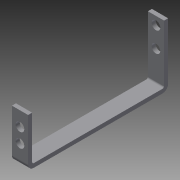
# Autodesk Inventor part: bottom pulley mount
Saved by Autodesk Inventor 2013 (Build 170138000, 138)
## iProperties
Created: 2013-02-07
Part Number: bottom pulley mount
Material: Generic
Document SubType Name: Sheet Metal
Designer: Arpan
Density: 1 g/cm^3
Sheet Metal Rule: Default
Mass: 7.12438 g
Surface Area: 60.3167 cm^2
Volume: 7.12438 cm^3
Author: Arpan
Autodesk Inventor part; units mm, degrees
ref_plane "YZ Plane" through (0, 0, 0) normal (1, 0, 0) x (0, 1, 0)
ref_plane "XZ Plane" through (0, 0, 0) normal (0, 1, 0) x (-1, 0, 0)
ref_plane "XY Plane" through (0, 0, 0) normal (0, 0, 1) x (1, 0, 0)
sketch "Sketch1" plane through (0, 0, 0) normal (0, 0, 1) x (1, 0, 0)
  line L0 (0, 0) -> (-12.7, 0)
  line L1 (-12.7, 0) -> (-12.7, 44.45)
  line L2 (-12.7, 44.45) -> (0, 44.45)
  line L3 (0, 44.45) -> (0, 0)
  dimension "d0" = 12.7
  dimension "d1" = 44.45
  measures "d0" distance of L0.start L0.end
  measures "d1" distance of L0.end L1.end
extrude "Plate1" add sketch "Sketch1" along normal blind 3.175
sketch "Sketch2" plane through (0, -1.27, 4.445) normal (0, -1, 0) x (1, 0, 0)
  line L0 (-12.7, 0) -> (0, 0)
  line L1 (0, 0) -> (0, 100.8952)
  line L2 (0, 100.8952) -> (-12.7, 100.8952)
  line L3 (-12.7, 100.8952) -> (-12.7, 0)
  constraints: 6 end point, 1 horizontal, 1 perpendicular, 1 vertical
edge flange "Flange1" height 105.3401 angle 90 thickness 3.175 bend radius 1.27 thickness toward (0, -1, 0) relief tear relief width 3.175 relief depth 1.5875 edges at (-6.35, 0, 3.175) wall of the first edge with corners at (-12.7, -1.27, 4.445) (0, -1.27, 4.445) (0, -1.27, 105.3401) (-12.7, -1.27, 105.3401)
bend "Bend1"
corner "Corner1"
sketch "Sketch3" plane through (0, 0, 0) normal (0, 0, -1) x (-1, 0, 0)
  circle A0 centre (6.3516, 38.1) radius 3.3782 projected
  circle A1 centre (6.3516, 22.225) radius 3.3782 projected
extrude "Cut1" cut sketch "Sketch3" against normal blind 3.175
sketch "Sketch5" plane through (0, 0, 106.6102) normal (0, 0, 1) x (1, 0, 0)
  line L0 (-12.7, 0) -> (0, 0)
  line L1 (0, 0) -> (0, 33.655)
  line L2 (0, 33.655) -> (-12.7, 33.655)
  line L3 (-12.7, 33.655) -> (-12.7, 0)
  constraints: 6 end point, 1 horizontal, 1 perpendicular, 1 vertical
edge flange "Flange2" height 38.1 angle 90 thickness 3.175 bend radius 1.27 thickness toward (0, 0, 1) relief tear relief width 3.175 relief depth 1.5875 edges at (-6.35, -1.27, 105.3401) wall of the first edge with corners at (-12.7, 0, 106.6102) (0, 0, 106.6102) (0, 33.655, 106.6102) (-12.7, 33.655, 106.6102)
bend "Bend2"
corner "Corner2"
sketch "Sketch6" plane through (-12.7, 33.655, 109.7851) normal (0, 0, 1) x (1, 0, 0)
  line L0 (0, 0) -> (12.7, 0) projected
  line L1 (0, -33.655) -> (0, 0) projected
  line L2 (6.35, 0) -> (6.35, -11.2183)
  line L3 (6.35, -11.2183) -> (6.35, -22.4451)
  circle A0 centre (6.35, -11.2183) radius 3.3782
  circle A1 centre (6.35, -22.4451) radius 3.3782
  dimension "d29" = 11.2183
  dimension "d31" = 11.2268
  dimension "d32" = 6.7564
  dimension "d33" = 6.7564
  constraints: 4 end point, 2 centre point, 2 coincident, 1 collinear, 1 midpoint, 1 parallel
  measures "d29" distance of L2.start L2.end
  measures "d31" distance of L2.end L3.end
  measures "d32" diameter of A0
  measures "d33" diameter of A1
extrude "Cut3" cut sketch "Sketch6" against normal blind 3.175
equation "\"d13\" = Thickness"
equation "\"d34\" = Thickness"
equation "\"d3\" = BendReliefWidth"
equation "\"d4\" = BendReliefDepth"
equation "\"d5\" = MinimumRemnant"
equation "\"d6\" = BendRadius"
equation "\"d10\" = CornerReliefSize"
equation "\"d11\" = GapSize"
equation "\"d12\" = JacobiRadiusSize"
equation "\"d19\" = BendReliefWidth"
equation "\"d20\" = BendReliefDepth"
equation "\"d21\" = MinimumRemnant"
equation "\"d22\" = BendRadius"
equation "\"d26\" = CornerReliefSize"
equation "\"d27\" = GapSize"
equation "\"d28\" = JacobiRadiusSize"
equation "\"BendRadius\" = Thickness"
equation "\"BendReliefWidth\" = Thickness"
equation "\"BendReliefDepth\" = 0.5 * Thickness"
equation "\"CornerReliefSize\" = 4 * Thickness"
equation "\"MinimumRemnant\" = 2 * Thickness"
equation "\"TransitionRadius\" = BendRadius"
equation "\"JacobiRadiusSize\" = Thickness"
equation "\"GapSize\" = Thickness"
equation "\"d2\" = BendRadius"
equation "\"Thickness\" = 3.175"
body "Solid1"
